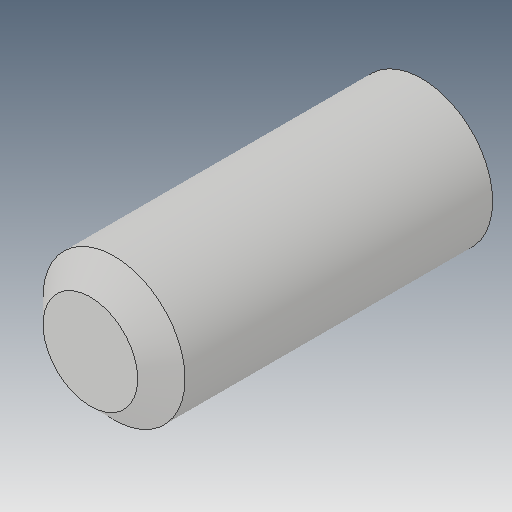
# Autodesk Inventor part: m3_setscrew
Saved by Autodesk Inventor 2020.3 (Build 243373000, 373)
## iProperties
Created: 2021-02-26
Part Number: m3_setscrew
Material: Generic
Document SubType Name: Modeling
Designer: paulg
Density: 1 g/cm^3
Appearance: Default
Author: paulg
Autodesk Inventor part; units mm, degrees
ref_plane "YZ Plane" through (0, 0, 0) normal (1, 0, 0) x (0, 1, 0)
ref_plane "XZ Plane" through (0, 0, 0) normal (0, 1, 0) x (-1, 0, 0)
ref_plane "XY Plane" through (0, 0, 0) normal (0, 0, 1) x (1, 0, 0)
sketch "Sketch1" plane through (0, 0, 0) normal (0, 0, 1) x (1, 0, 0)
  circle A0 centre (0, 0) radius 1.5
  dimension "d0" = 3
  constraints: 1 centre point, 1 coincident
  measures "d0" diameter of A0
extrude "Extrusion1" add sketch "Sketch1" along normal blind 7
chamfer "Chamfer1" distance 0.5 angle 45 1 edges at (-1.5, 0, 7)
sketch "Sketch2" plane through (0, 0, 0) normal (0, 0, -1) x (-1, 0, 0)
  line L0 (-0.5196, 0.9) -> (0.5196, 0.9)
  line L1 (0.5196, 0.9) -> (1.0392, 0)
  line L2 (1.0392, 0) -> (0.5196, -0.9)
  line L3 (0.5196, -0.9) -> (-0.5196, -0.9)
  line L4 (-0.5196, -0.9) -> (-1.0392, 0)
  line L5 (-1.0392, 0) -> (-0.5196, 0.9)
  point P0 (0, 0)
  point P1 (0, 0)
  dimension "d6" = 1.8
  constraints: 12 end point, 1 coincident, 1 horizontal, 13 other
  measures "d6" distance between parallel lines of L3 L0
extrude "Extrusion2" cut sketch "Sketch2" against normal blind 2
body "Solid1"
